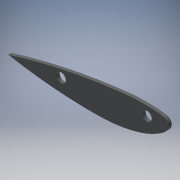
# Autodesk Inventor part: plate
Saved by Autodesk Inventor 2018.2 (Build 222227000, 227)
## iProperties
Created: 2018-03-05
Part Number: plate
Material: 木材 (オーク)
Document SubType Name: Modeling
Designer: ku_sk
Density: 0.76 g/cm^3
Appearance: ホワイト オーク材 - ナチュラル 標準の光沢
Author: ku_sk
Autodesk Inventor part; units mm, degrees
ref_plane "YZ Plane" through (0, 0, 0) normal (1, 0, 0) x (0, 1, 0)
ref_plane "XZ Plane" through (0, 0, 0) normal (0, 1, 0) x (-1, 0, 0)
ref_plane "XY Plane" through (0, 0, 0) normal (0, 0, 1) x (1, 0, 0)
sketch "スケッチ1" plane through (0, 0, 0) normal (0, 1, 0) x (-1, 0, 0)
  arc A0 (209.8798, -23.6971) -> (38.3003, 12.1023) centre (-36.3979, -774.9853) ccw projected
  arc A1 (99.4686, -35.9265) -> (209.8798, -23.6971) centre (88.5018, 567.6156) ccw projected
  arc A2 (73.7238, -35.6322) -> (99.4686, -35.9265) centre (91.566, 398.982) ccw projected
  arc A3 (26.4399, -27.2272) -> (73.7238, -35.6322) centre (81.048, 142.776) ccw projected
  arc A4 (-0.8557, -13.8205) -> (26.4399, -27.2272) centre (58.458, 72.45) ccw projected
  arc A5 (-8.6045, -6.2961) -> (-0.8557, -13.8205) centre (17.4, 12.732) ccw projected
  arc A6 (-1.8835, 10.4943) -> (-8.6045, -6.2961) centre (0, 0) ccw projected
  arc A7 (18.284, 12.3227) -> (-1.8835, 10.4943) centre (18.66, -103.968) ccw projected
  arc A8 (38.3003, 12.1023) -> (18.284, 12.3227) centre (20.556, -690.396) ccw projected
extrude "押し出し1" add sketch "スケッチ1" along normal blind 4
sketch "スケッチ2" plane through (0, 0, 0) normal (0, -1, 0) x (1, 0, 0)
  circle A0 centre (-20, -2.2582) radius 6
  circle A1 centre (-130, -14.678) radius 6
  line L0 (0, 0) -> (-209.8798, -23.6971)
  dimension "d3" = 12
  dimension "d4" = 12
  dimension "d5" = 20
  dimension "d6" = 130
  constraints: 2 centre point, 2 end point, 2 point on line
  measures "d3" diameter of A0
  measures "d4" diameter of A1
  measures "d5" horizontal distance of L0.start A0.centre
  measures "d6" horizontal distance of A1.centre L0.start
extrude "押し出し2" cut sketch "スケッチ2" against normal through all
thicken "厚み1" operation cut thickness 3 both sides no extend neighbours no toward (0.2114907, 0, -0.97738) faces at (-130.8117, 2.6667, -2.245) (-36.0766, 2.6667, 12.1549) (-0.3377, 1.3333, 10.8708) (9.052, 1.3333, -5.6337) (1.8363, 1.3333, -13.1189) (-10.787, 2.6667, -20.7604) (-68.3801, 1.3333, -35.3326) (-85.1636, 2.6667, -35.9512) (-200.7848, 1.3333, -25.4914)
equation "\"d4\" = d3"
